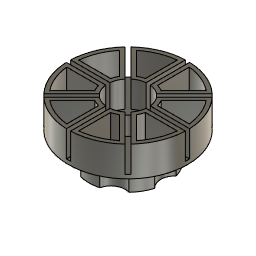
Giunto accoppiamento motore ruota v3 (Autodesk Fusion 360 design; units mm, degrees)
Autodesk Fusion 360 part; units mm, degrees
note: some values were not read from the file. Set by a fixed rule: which face or edge a step refers to.
sketch "Schizzo1" plane through (0, 0, 0) normal (0, 0, 1) x (1, 0, 0)
  circle A0 centre (0, 0) radius 29.75
  circle A1 centre (0, 0) radius 25 construction
  circle A2 centre (35.9948, 0) radius 10.9948
  line L0 (0, 0) -> (17.9974, 31.1724) construction
  line L1 (0, 0) -> (35.9948, 0) construction
  circle A3 centre (17.9974, 31.1724) radius 10.9948
  line L2 (21.3625, 20.7052) -> (28.6125, 8.1479) construction
  circle A4 centre (-17.9974, 31.1724) radius 10.9948
  circle A5 centre (-35.9948, 0) radius 10.9948
  circle A6 centre (-17.9974, -31.1724) radius 10.9948
  circle A7 centre (17.9974, -31.1724) radius 10.9948
  dimension "d1" = 59.5
  dimension "d2" = 50
  dimension "d3" = 60
  dimension "d4" = 14.5
  dimension "d6" = 360
  constraint coincident A0.centre A1.centre
  constraint tangent A1 A2
  constraint coincident A2.centre L1.end
  constraint horizontal L1
  constraint equal L0 L1
  constraint coincident L0.end A3.centre
  constraint equal A2 A3
  constraint coincident A0 L2.start
  constraint coincident A3 L2.start
  constraint coincident A2 L2.end
  constraint coincident A0 L2.end
  measures "d1" diameter of A0
  measures "d2" diameter of A1
  measures "d3" angle of L0 L1
  measures "d4" distance of L2.start L2.end
extrude "Estrusione1" add sketch "Schizzo1" along normal blind 20 contours A0 A2 A3 A4 A5 A6 A7 makes body 1
sketch "Schizzo2" plane through (0, 0, 20) normal (0, 0, 1) x (-1, 0, 0)
  arc A0 (28.6125, 8.1479) -> (21.3625, 20.7052) centre (0, 0) ccw
  arc A1 (7.25, 28.8531) -> (21.3625, 20.7052) centre (17.9974, 31.1724) ccw
  arc A2 (7.25, 28.8531) -> (-7.25, 28.8531) centre (0, 0) ccw
  arc A3 (-21.3625, 20.7052) -> (-7.25, 28.8531) centre (-17.9974, 31.1724) ccw
  arc A4 (-21.3625, 20.7052) -> (-28.6125, 8.1479) centre (0, 0) ccw
  arc A5 (-28.6125, -8.1479) -> (-28.6125, 8.1479) centre (-35.9948, 0) ccw
  arc A6 (-28.6125, -8.1479) -> (-21.3625, -20.7052) centre (0, 0) ccw
  arc A7 (-7.25, -28.8531) -> (-21.3625, -20.7052) centre (-17.9974, -31.1724) ccw
  arc A8 (-7.25, -28.8531) -> (7.25, -28.8531) centre (0, 0) ccw
  arc A9 (21.3625, -20.7052) -> (7.25, -28.8531) centre (17.9974, -31.1724) ccw
  arc A10 (21.3625, -20.7052) -> (28.6125, -8.1479) centre (0, 0) ccw
  arc A11 (28.6125, 8.1479) -> (28.6125, -8.1479) centre (35.9948, 0) ccw
  circle A12 centre (0, 0) radius 45.5
  circle A13 centre (0, 0) radius 15.5
  dimension "d9" = 91
  dimension "d10" = 31
  constraint coincident A0.centre A2.centre
  measures "d9" diameter of A12
  measures "d10" diameter of A13
extrude "Estrusione2" add sketch "Schizzo2" along normal blind 23 contours A0 A1 A2 A3 A4 A5 A6 A7 A8 A9 A10 A11 | A12 bodies 1
sketch "Schizzo3" plane through (0, 0, 43) normal (0, 0, 1) x (-1, 0, 0)
  circle A0 centre (0, 0) radius 15.5
  circle A1 centre (0, 0) radius 45.5
  line L0 (-1.6, 93.0019) -> (1.6, 93.0019)
  line L1 (1.6, 93.0019) -> (1.6, 6.4)
  line L2 (1.6, 6.4) -> (-1.6, 6.4)
  line L3 (-1.6, 6.4) -> (-1.6, 93.0019)
  line L4 (-1.6, 6.4) -> (0, 0) construction
  line L5 (0, 0) -> (1.6, 6.4) construction
  dimension "d13" = 3.2
  constraint horizontal L0
  constraint vertical L1
  constraint horizontal L2
  constraint vertical L3
  constraint coincident A0.centre A1.centre
  constraint equal L4 L5
  measures "d13" distance of L0.start L0.end
extrude "Estrusione3" cut sketch "Schizzo3" against normal up to surface (20 mm away) contours A0 A1 L1 L3 picked at (0.1778, 25.4928) bodies 1
pattern_circular "Serie C1" count 8 over 360 about axis through (0, 0, 20) along (0, 0, 1) of "Estrusione3"
sketch "Schizzo4" plane through (0, 0, 0) normal (0, 0, -1) x (1, 0, 0)
  arc A0 (-21.3625, 20.7052) -> (-28.6125, 8.1479) centre (0, 0) ccw
  arc A1 (-28.6125, -8.1479) -> (-28.6125, 8.1479) centre (-35.9948, 0) ccw
  arc A2 (-28.6125, -8.1479) -> (-21.3625, -20.7052) centre (0, 0) ccw
  arc A3 (-7.25, -28.8531) -> (-21.3625, -20.7052) centre (-17.9974, -31.1724) ccw
  arc A4 (-7.25, -28.8531) -> (7.25, -28.8531) centre (0, 0) ccw
  arc A5 (21.3625, -20.7052) -> (7.25, -28.8531) centre (17.9974, -31.1724) ccw
  arc A6 (21.3625, -20.7052) -> (28.6125, -8.1479) centre (0, 0) ccw
  arc A7 (28.6125, 8.1479) -> (28.6125, -8.1479) centre (35.9948, 0) ccw
  arc A8 (28.6125, 8.1479) -> (21.3625, 20.7052) centre (0, 0) ccw
  arc A9 (7.25, 28.8531) -> (21.3625, 20.7052) centre (17.9974, 31.1724) ccw
  arc A10 (7.25, 28.8531) -> (-7.25, 28.8531) centre (0, 0) ccw
  arc A11 (-21.3625, 20.7052) -> (-7.25, 28.8531) centre (-17.9974, 31.1724) ccw
  circle A12 centre (0, 0) radius 10
  dimension "d18" = 20
  constraint coincident A0.centre A2.centre
  measures "d18" diameter of A12
extrude "Estrusione4" cut sketch "Schizzo4" against normal through all contours A12 bodies 1
sketch "Schizzo5" plane through (0, 0, 43) normal (0, 0, 1) x (-1, 0, 0)
  line L0 (31.0221, -33.2848) -> (9.7702, -12.033)
  arc A0 (1.6, -15.4172) -> (9.7702, -12.033) centre (0, 0) ccw
  line L1 (1.6, -15.4172) -> (1.6, -45.4719)
  arc A1 (1.6, -45.4719) -> (31.0221, -33.2848) centre (0, 0) ccw
  line L2 (26.6228, -33.1282) -> (9.4179, -15.9233)
  arc A2 (4.6, -17.919) -> (9.4179, -15.9233) centre (0, 0) ccw
  line L3 (4.6, -17.919) -> (4.6, -42.2503)
  arc A3 (4.6, -42.2503) -> (26.6228, -33.1282) centre (0, 0) ccw
  dimension "d20" = 3
extrude "Estrusione5" cut sketch "Schizzo5" against normal up to surface (20 mm away) contours L2 A2 L3 A3 bodies 1
pattern_circular "Serie C2" count 8 over 360 about axis through (0, 0, 20) along (0, 0, 1) of "Estrusione5"
sketch "Schizzo6" plane through (0, 0, 0) normal (0, 0, -1) x (1, 0, 0)
  circle A0 centre (0, 0) radius 10
  arc A1 (-21.3625, 20.7052) -> (-28.6125, 8.1479) centre (0, 0) ccw
  arc A2 (-28.6125, -8.1479) -> (-28.6125, 8.1479) centre (-35.9948, 0) ccw
  arc A3 (-28.6125, -8.1479) -> (-21.3625, -20.7052) centre (0, 0) ccw
  arc A4 (-7.25, -28.8531) -> (-21.3625, -20.7052) centre (-17.9974, -31.1724) ccw
  arc A5 (-7.25, -28.8531) -> (7.25, -28.8531) centre (0, 0) ccw
  arc A6 (21.3625, -20.7052) -> (7.25, -28.8531) centre (17.9974, -31.1724) ccw
  arc A7 (21.3625, -20.7052) -> (28.6125, -8.1479) centre (0, 0) ccw
  arc A8 (28.6125, 8.1479) -> (28.6125, -8.1479) centre (35.9948, 0) ccw
  arc A9 (28.6125, 8.1479) -> (21.3625, 20.7052) centre (0, 0) ccw
  arc A10 (7.25, 28.8531) -> (21.3625, 20.7052) centre (17.9974, 31.1724) ccw
  arc A11 (7.25, 28.8531) -> (-7.25, 28.8531) centre (0, 0) ccw
  arc A12 (-21.3625, 20.7052) -> (-7.25, 28.8531) centre (-17.9974, 31.1724) ccw
  arc A13 (4.8776, 26.3016) -> (-4.8776, 26.3016) centre (0, 0) ccw
  arc A14 (-20.339, 17.3749) -> (-4.8776, 26.3016) centre (-17.9974, 31.1724) ccw
  arc A15 (-20.339, 17.3749) -> (-25.2166, 8.9267) centre (0, 0) ccw
  arc A16 (-25.2166, -8.9267) -> (-25.2166, 8.9267) centre (-35.9948, 0) ccw
  arc A17 (-25.2166, -8.9267) -> (-20.339, -17.3749) centre (0, 0) ccw
  arc A18 (-4.8776, -26.3016) -> (-20.339, -17.3749) centre (-17.9974, -31.1724) ccw
  arc A19 (-4.8776, -26.3016) -> (4.8776, -26.3016) centre (0, 0) ccw
  arc A20 (20.339, -17.3749) -> (4.8776, -26.3016) centre (17.9974, -31.1724) ccw
  arc A21 (20.339, -17.3749) -> (25.2166, -8.9267) centre (0, 0) ccw
  arc A22 (25.2166, 8.9267) -> (25.2166, -8.9267) centre (35.9948, 0) ccw
  arc A23 (25.2166, 8.9267) -> (20.339, 17.3749) centre (0, 0) ccw
  arc A24 (4.8776, 26.3016) -> (20.339, 17.3749) centre (17.9974, 31.1724) ccw
  circle A25 centre (0, 0) radius 13
  dimension "d25" = 3
  dimension "d26" = 3
extrude "Estrusione6" cut sketch "Schizzo6" against normal up to surface (20 mm away) contours A13 A14 A15 A16 A17 A18 A19 A20 A21 A22 A23 A24 bodies 1 makes body 2 at (12.9838, 0.648, 13.3333)
sketch "Schizzo7" plane through (0, 0, 20) normal (0, 0, 1) x (-1, 0, 0)
  circle A0 centre (0, 0) radius 13
  circle A1 centre (0, 0) radius 10
  circle A2 centre (0, 0) radius 10
  circle A3 centre (0, 0) radius 15.5
  arc A4 (-12.033, 9.7702) -> (-15.4172, 1.6) centre (0, 0) ccw
  constraint coincident A0.centre A1.centre
  constraint equal A1 A2
  constraint concentric A2 A3
  constraint equal A3 A4
extrude "Estrusione7" add sketch "Schizzo7" along normal up to surface (3 mm away) contours A0 | A3 A4 bodies 1 2
equation "d3 = ( 360 / 6 ) * 1 deg"
